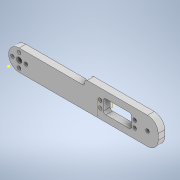
# Autodesk Inventor part: Claw arm
Saved by Autodesk Inventor 2020 (Build 240168000, 168)
## iProperties
Created: 2020-01-21
Part Number: Claw arm
Material: Generic
Document SubType Name: Modeling
Designer: ian.golightly
Density: 1 g/cm^3
Appearance: Default
Author: ian.golightly
Autodesk Inventor part; units mm, degrees
ref_plane "YZ Plane" through (0, 0, 0) normal (1, 0, 0) x (0, 1, 0)
ref_plane "XZ Plane" through (0, 0, 0) normal (0, 1, 0) x (-1, 0, 0)
ref_plane "XY Plane" through (0, 0, 0) normal (0, 0, 1) x (1, 0, 0)
sketch "Sketch1" plane through (0, 0, 0) normal (0, 0, 1) x (1, 0, 0)
  point P0 (0, 0)
sketch "Sketch2" plane through (0, 0, 0) normal (0, 0, 1) x (1, 0, 0)
  line L0 (0, 0) -> (215.9, 0)
  line L1 (215.9, 0) -> (215.9, 50.8)
  line L2 (215.9, 50.8) -> (0, 50.8)
  line L3 (0, 50.8) -> (0, 0)
  dimension "d0" = 215.9
  dimension "d1" = 50.8
  constraints: 8 end point, 2 parallel, 1 horizontal, 1 perpendicular
  measures "d0" distance of L2.end L1.end
  measures "d1" distance of L1.end L0.end
extrude "Extrusion1" add sketch "Sketch2" along normal blind 9.525
sketch "Sketch3" plane through (0, 0, 9.525) normal (0, 0, 1) x (1, 0, 0)
  line L0 (215.9, 0) -> (215.9, 50.8) projected
  line L1 (215.9, 0) -> (215.9, 30.48)
  line L2 (0, 0) -> (0, 30.48)
  line L3 (0, 50.8) -> (0, 0) projected
  line L4 (0, 30.48) -> (215.9, 30.48)
  line L5 (215.9, 0) -> (203.2, 0)
  line L6 (0, 0) -> (215.9, 0) projected
  line L7 (203.2, 0) -> (203.2, 50.8)
  line L8 (215.9, 50.8) -> (0, 50.8) projected
  line L9 (203.2, 0) -> (177.8, 0)
  line L10 (177.8, 0) -> (152.4, 0)
  line L11 (177.8, 0) -> (137.16, 0)
  line L12 (177.8, 0) -> (177.8, 9.525)
  line L13 (177.8, 9.525) -> (137.16, 9.525)
  line L14 (137.16, 9.525) -> (177.8, 9.525)
  line L15 (177.8, 9.525) -> (177.8, 30.48)
  line L16 (177.8, 30.48) -> (137.16, 30.48)
  line L17 (137.16, 30.48) -> (137.16, 9.525)
  line L18 (137.16, 9.525) -> (177.36, 9.525)
  line L19 (177.36, 9.525) -> (177.36, 29.525)
  line L20 (177.36, 29.525) -> (137.16, 29.525)
  line L21 (137.16, 29.525) -> (137.16, 9.525)
  point P0 (177.36, 9.525)
  dimension "d4" = 30.48
  dimension "d5" = 30.48
  dimension "d6" = 12.7
  dimension "d7" = 25.4
  dimension "d8" = 25.4
  dimension "d9" = 40.64
  dimension "d10" = 9.525
  dimension "d11" = 40.64
  dimension "d12" = 40.2
  dimension "d13" = 20
  constraints: 36 end point, 8 point on line, 4 parallel, 4 perpendicular, 2 horizontal, 1 vertical
  measures "d4" distance of L0.start L1.end
  measures "d5" distance of L2.start L2.end
  measures "d6" distance of L0.start L5.end
  measures "d7" distance of L5.end L9.end
  measures "d8" distance of L9.end L10.end
  measures "d9" distance of L9.end L11.end
  measures "d10" distance of L9.end L12.end
  measures "d11" distance of L12.end L13.end
  measures "d12" distance of L20.end L19.end
  measures "d13" distance of L19.end L18.end
extrude "Extrusion2" cut sketch "Sketch3" against normal blind 25.4 contours L13 L17 L20 L19
sketch "Sketch4" plane through (0, 0, 9.525) normal (0, 0, 1) x (1, 0, 0)
  line L0 (0, 0) -> (0, 30.48)
  line L1 (0, 50.8) -> (0, 0) projected
  line L2 (137.16, 29.525) -> (177.36, 29.525) projected
  line L3 (0, 30.48) -> (137.16, 29.525)
  line L4 (215.9, 50.8) -> (0, 50.8) projected
  line L5 (0, 30.48) -> (111.76, 30.48)
  line L6 (111.76, 30.48) -> (111.76, 50.8)
  line L7 (111.76, 50.8) -> (0, 50.8)
  line L8 (0, 50.8) -> (0, 30.48)
  arc A0 (111.76, 40.64) -> (109.4345, 29.525) centre (137.16, 29.525) ccw
  point P0 (109.451, 30.48)
  dimension "d16" = 30.48
  constraints: 12 end point, 2 parallel, 2 point on circle, 2 point on line, 1 centre point, 1 coincident, 1 horizontal, 1 midpoint, 1 perpendicular
  measures "d16" distance of L0.start L0.end
extrude "Extrusion3" cut sketch "Sketch4" against normal blind 25.4 contours L4 L6 A0 L5 L1
sketch "Sketch5" plane through (0, 0, 9.525) normal (0, 0, 1) x (1, 0, 0)
  line L0 (137.16, 9.525) -> (177.36, 9.525) projected
  line L1 (137.16, 9.525) -> (132.36, 9.525)
  line L2 (132.36, 9.525) -> (132.36, 13.9192)
  circle A0 centre (132.36, 13.9192) radius 2.25
  line L3 (132.36, 13.9192) -> (132.36, 23.8192)
  circle A1 centre (132.36, 23.8192) radius 2.2479
  line L4 (177.36, 9.525) -> (182.1606, 9.525)
  line L5 (182.1606, 9.525) -> (182.1606, 13.9192)
  circle A2 centre (182.1606, 13.9192) radius 2.2479
  line L6 (182.1606, 13.9192) -> (182.1606, 23.8252)
  circle A3 centre (182.1606, 23.8252) radius 2.2479
  point P0 (0, 0)
  dimension "d19" = 4.8
  dimension "d20" = 4.3942
  dimension "d21" = 4.5
  dimension "d22" = 9.9
  dimension "d23" = 4.4958
  dimension "d24" = 4.8006
  dimension "d25" = 4.3942
  dimension "d26" = 4.4958
  dimension "d27" = 9.906
  dimension "d28" = 4.4958
  constraints: 12 end point, 4 centre point, 4 coincident, 3 vertical, 2 horizontal, 1 perpendicular
  measures "d19" distance of L0.start L1.end
  measures "d20" distance of L1.end L2.end
  measures "d21" diameter of A0
  measures "d22" distance of L3.start L3.end
  measures "d23" diameter of A1
  measures "d24" distance of L0.end L4.end
  measures "d25" distance of L4.end L5.end
  measures "d26" diameter of A2
  measures "d27" distance of L6.start L6.end
  measures "d28" diameter of A3
extrude "Extrusion4" cut sketch "Sketch5" against normal blind 25.4
sketch "Sketch7" plane through (0, 0, 9.525) normal (0, 0, 1) x (1, 0, 0)
  line L0 (177.36, 29.525) -> (177.36, 9.525) projected
  line L1 (177.36, 9.525) -> (215.9, 9.525)
  line L2 (215.9, 0) -> (215.9, 50.8) projected
  circle A0 centre (182.1606, 13.9192) radius 2.2479 projected
  line L3 (184.4085, 13.9192) -> (215.9, 13.9192)
  line L4 (175.586, 50.8) -> (175.586, 0)
  line L5 (0, 0) -> (215.9, 0) projected
  line L6 (141.0803, 19.525) -> (205.5055, 19.525)
  circle A1 centre (175.586, 19.525) radius 2.2479
  dimension "d33" = 4.4958
  constraints: 8 end point, 4 point on line, 3 horizontal, 1 centre point, 1 horizontal alignment, 1 vertical, 1 other
  measures "d33" diameter of A1
extrude "Extrusion6" cut sketch "Sketch7" against normal blind 25.4 contours A1 L6 L0 | L0 L6 L4 A1 | L6 A1 L0 | L0 A1 L4 L6 | L4 L6 A1 | L4 A1 L6
sketch "Sketch8" plane through (0, 0, 9.525) normal (0, 0, 1) x (1, 0, 0)
  point P0 (0, 0)
sketch "Sketch9" plane through (0, 0, 9.525) normal (0, 0, 1) x (1, 0, 0)
  point P0 (0, 0)
sketch "Sketch10" plane through (0, 0, 9.525) normal (0, 0, 1) x (1, 0, 0)
  point P0 (0, 0)
fillet "Fillet1" radius 3.175 4 edges at (137.16, 9.525, 4.7625) (137.16, 29.525, 4.7625) (177.36, 29.525, 4.7625) (177.36, 9.525, 4.7625)
fillet "Fillet2" radius 3.175 3 edges at (111.76, 50.8, 4.7625) (111.76, 40.64, 4.7625) (109.451, 30.48, 4.7625)
fillet "Fillet3" radius 15.24 4 edges at (0, 30.48, 4.7625) (0, 0, 4.7625) (215.9, 50.8, 4.7625) (215.9, 0, 4.7625)
sketch "Sketch11" plane through (0, 0, 9.525) normal (0, 0, 1) x (1, 0, 0)
  line L0 (106.5367, 30.48) -> (15.24, 30.48) projected
  line L1 (15.24, 0) -> (200.66, 0) projected
  line L2 (15.24, 30.48) -> (15.24, 0)
  line L3 (15.24, 0) -> (15.24, 15.24)
  line L4 (15.24, 15.24) -> (30.48, 15.24)
  line L5 (30.48, 15.24) -> (0, 15.24)
  arc A0 (15.24, 30.48) -> (15.24, 0) centre (15.24, 15.24) ccw projected
  circle A1 centre (15.24, 15.24) radius 3.81
  circle A2 centre (25.019, 15.24) radius 1.3589
  circle A3 centre (15.24, 25.019) radius 1.3589
  circle A4 centre (5.461, 15.24) radius 1.3589
  circle A5 centre (15.24, 5.461) radius 1.3589
  point P0 (0, 0)
  dimension "d39" = 15.24
  dimension "d40" = 7.62
  dimension "d41" = 2.7178
  dimension "d42" = 2.7178
  dimension "d43" = 2.7178
  dimension "d44" = 2.7178
  constraints: 8 end point, 5 centre point, 4 point on line, 1 coincident, 1 horizontal, 1 midpoint, 1 point on circle, 1 vertical
  measures "d39" distance of L3.end L4.end
  measures "d40" diameter of A1
  measures "d41" diameter of A2
  measures "d42" diameter of A3
  measures "d43" diameter of A4
  measures "d44" diameter of A5
extrude "Extrusion7" cut sketch "Sketch11" against normal blind 25.4 contours A2 L4 | L4 A2 | A3 L2 | L2 A3 | A4 L5 | L5 A4 | A1 L4 L2 | L2 L5 A1 | A5 L2 | L2 A5 | L4 A1 L2 | L2 A1 L5
sketch "Sketch12" plane through (0, 0, 9.525) normal (0, 0, 1) x (1, 0, 0)
  circle A0 centre (5.461, 15.24) radius 1.3589 projected
  circle A1 centre (5.461, 15.24) radius 2.2479
  circle A2 centre (15.24, 5.461) radius 1.3589 projected
  circle A3 centre (15.24, 5.461) radius 2.2479
  circle A4 centre (25.019, 15.24) radius 1.3589 projected
  circle A5 centre (25.019, 15.24) radius 2.2479
  circle A6 centre (15.24, 25.019) radius 1.3589 projected
  circle A7 centre (15.24, 25.019) radius 2.2479
  circle A8 centre (15.24, 25.019) radius 2.54
  circle A9 centre (25.019, 15.24) radius 2.54
  circle A10 centre (5.461, 15.24) radius 2.54
  circle A11 centre (15.24, 5.461) radius 2.54
  circle A12 centre (132.36, 13.9192) radius 2.25 projected
  circle A13 centre (132.36, 13.9192) radius 2.54
  circle A14 centre (132.36, 23.8192) radius 2.2479 projected
  circle A15 centre (132.36, 23.8192) radius 2.54
  circle A16 centre (182.1606, 23.8252) radius 2.2479 projected
  circle A17 centre (182.1606, 23.8252) radius 2.54
  circle A18 centre (182.1606, 13.9192) radius 2.2479 projected
  circle A19 centre (182.1606, 13.9192) radius 2.54
  arc A20 (177.36, 18.1445) -> (177.36, 20.9055) centre (175.586, 19.525) ccw projected
  circle A21 centre (175.586, 19.525) radius 2.54
  point P0 (0, 0)
  dimension "d47" = 4.4958
  dimension "d48" = 4.4958
  dimension "d49" = 4.4958
  dimension "d50" = 4.4958
  dimension "d51" = 5.08
  dimension "d52" = 5.08
  dimension "d53" = 5.08
  dimension "d54" = 5.08
  dimension "d55" = 5.08
  dimension "d56" = 5.08
  dimension "d57" = 5.08
  dimension "d58" = 5.08
  dimension "d59" = 5.08
  constraints: 13 centre point, 13 coincident
  measures "d47" diameter of A1
  measures "d48" diameter of A3
  measures "d49" diameter of A5
  measures "d50" diameter of A7
  measures "d51" diameter of A8
  measures "d52" diameter of A9
  measures "d53" diameter of A10
  measures "d54" diameter of A11
  measures "d55" diameter of A13
  measures "d56" diameter of A15
  measures "d57" diameter of A17
  measures "d58" diameter of A19
  measures "d59" diameter of A21
extrude "Extrusion8" cut sketch "Sketch12" against normal blind 25.4 contours A0 | A1 | A2 | A3 | A4 | A5 | A6 | A7 | A8 | A9 | A10 | A11 | A12 | A13 | A14 | A15 | A16 | A17 | A18 | A19 | A21
sketch "Sketch13" plane through (0, 0, 9.525) normal (0, 0, 1) x (1, 0, 0)
  point P0 (0, 0)
ref_plane "Work Plane1" through (129.9559, 14.7389, 0) normal (1, 0, 0) x (0, 0, -1)
sketch "Sketch14" plane through (129.9559, 14.7389, 0) normal (1, 0, 0) x (0, 0, -1)
  point P0 (0, -14.7389)
sketch "Sketch15" plane through (0, 0, 0) normal (0, 0, -1) x (-1, 0, 0)
  line L0 (-160.2621, 50.5435) -> (-160.2621, 29.525)
  line L1 (-174.185, 29.525) -> (-140.335, 29.525) projected
  line L2 (-156.9844, 29.525) -> (-156.9844, 39.05)
  line L3 (-109.6833, 39.05) -> (-217.5289, 39.05)
  line L4 (-217.5289, 39.05) -> (-217.5289, 53.1054)
  line L5 (-217.5289, 53.1054) -> (-109.6833, 53.1054)
  line L6 (-109.6833, 53.1054) -> (-109.6833, 39.05)
  point P0 (0, 0)
  point P1 (-184.6931, 29.525)
  point P2 (-129.9559, 29.525)
  dimension "d62" = 9.525
  constraints: 12 end point, 3 parallel, 2 point on line, 1 horizontal, 1 perpendicular, 1 vertical
  measures "d62" distance of L2.start L2.end
extrude "Extrusion9" cut sketch "Sketch15" against normal blind 25.4 contours L3 L4 L5 L6
fillet "Fillet4" radius 15.24 1 edges at (215.4951, 39.05, 4.7625)
fillet "Fillet5" radius 3.175 1 edges at (111.122, 39.05, 4.7625)
sketch "Sketch16" plane through (0, 0, 9.525) normal (0, 0, 1) x (1, 0, 0)
  line L0 (215.9, 15.24) -> (215.9, 23.81) projected
  line L1 (215.9, 19.525) -> (178.126, 19.525)
  arc A0 (177.36, 17.7072) -> (177.36, 21.3428) centre (175.586, 19.525) ccw projected
  arc A1 (200.66, 0) -> (215.9, 15.24) centre (200.66, 15.24) ccw projected
  line L2 (113.4449, 39.05) -> (200.66, 39.05) projected
  line L3 (200.66, 0) -> (200.66, 39.05)
  circle A2 centre (200.66, 19.525) radius 2.54
  point P0 (0, 0)
  dimension "d68" = 5.08
  constraints: 4 end point, 2 midpoint, 1 centre point, 1 horizontal, 1 point on circle, 1 vertical
  measures "d68" diameter of A2
extrude "Extrusion10" cut sketch "Sketch16" against normal blind 25.4 contours A2 L3 L1 | L1 L3 A2 | A2 L1 L3 | L1 A2 L3
body "Solid1"
